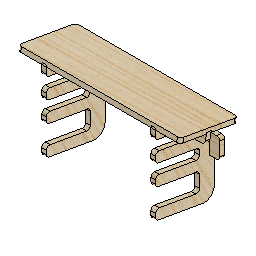
model (Autodesk Fusion 360 design; units mm, degrees)
Autodesk Fusion 360 part; units mm, degrees
note: some values were not read from the file. Set by a fixed rule: which sketch regions a step uses.
sketch "side" plane through (0, 0, 0) normal (1, 0, 0) x (0, 1, 0) in component "mount"
  line L0 (0, 0) -> (0, 102.8022)
  line L1 (0, 102.8022) -> (-75.1927, 116.0607)
  line L2 (-75.1927, 116.0607) -> (-75.1927, 102.8601)
  line L3 (-75.1927, 102.8601) -> (-19, 92.9519)
  line L4 (-19, 92.9519) -> (-19, 79.9519)
  line L5 (-19, 79.9519) -> (-75.1927, 89.8601)
  line L6 (-75.1927, 89.8601) -> (-75.1927, 76.6596)
  line L7 (-75.1927, 76.6596) -> (-19, 66.7513)
  line L8 (-19, 66.7513) -> (-19, 53.7513)
  line L9 (-19, 53.7513) -> (-75.1927, 63.6596)
  line L10 (-75.1927, 63.6596) -> (-75.1927, 50.459)
  line L11 (-75.1927, 50.459) -> (-19, 40.5508)
  line L12 (-19, 40.5508) -> (-19, 16.5508)
  line L13 (-19, 16.5508) -> (-75.1927, 26.459)
  line L14 (-75.1927, 26.459) -> (-75.1927, 13.2585)
  line L15 (-75.1927, 13.2585) -> (0, 0)
  line L16 (-19, 92.9519) -> (0, 92.9519) construction
  line L17 (-74.8454, 115.9994) -> (-75.1927, 114.0298)
  line L18 (-74.8454, 115.9994) -> (-74.1508, 119.9387) construction
  line L19 (-75.1927, 116.0607) -> (-75.1927, 119.9387) construction
  line L20 (-74.1508, 119.9387) -> (-75.1927, 119.9387) construction
  dimension "d9" = 80
  dimension "d14" = 13
  dimension "d15" = 13
  dimension "d16" = 13
  dimension "d21" = 2
  dimension "d33" = 24
  dimension "d43" = 4
  dimension "d44" = 76
  dimension "d53" = 19
  constraint coincident L0.start L15.end
  constraint vertical L0
  constraint parallel L0 L2
  constraint parallel L1 L3
  constraint parallel L0 L4
  constraint coincident L0 L16.end
  constraint perpendicular L0 L16
  constraint collinear L2 L6
  constraint collinear L6 L10
  constraint collinear L10 L14
  constraint collinear L4 L8
  constraint collinear L8 L12
  constraint equal L2 L6
  constraint equal L6 L10
  constraint equal L10 L14
  constraint parallel L5 L7
  constraint parallel L9 L11
  constraint parallel L13 L15
  constraint parallel L3 L5
  constraint parallel L7 L9
  constraint parallel L11 L13
  constraint coincident L1 L17.start
  constraint coincident L2 L17.end
  constraint perpendicular L1 L17
  constraint perpendicular L1 L18
  constraint parallel L2 L19
  constraint perpendicular L19 L20
  measures "d9" angle of L0 L1
  measures "d14" distance of L3.end L4.end
  measures "d15" distance of L1 L3
  measures "d16" distance of L7.end L8.end
  measures "d21" distance of L17.start L17.end
  measures "d33" distance of L11.end L12.end
  measures "d43" distance of L17.start L18.end
  measures "d44" distance of L0.end L17.start
  measures "d53" distance of L0 L4
extrude "Extrude1" add sketch "side" along normal blind 6 contours L0 L1 L2 L3 L4 L5 L6 L7 L8 L9 L10 L11 L12 L13 L14 L15 L17 makes body 1 in component "mount"
copy_body "CopyPasteBodies1" bodies 1 makes body 2 in component "mount"
move_body "Move1" bodies 2 to x (1, 0, 0) y (0, 1, 0) z (0, 0, 1) at (140, 0, 0) in component "mount"
sketch "top" plane through (0, 17.5802, 99.7023) normal (0, 0.173648, 0.984808) x (-1, 0, 0) in component "mount"
  line L0 (0, 17.8514) -> (0, 93.8514)
  line L1 (0, 93.8514) -> (-6, 93.8514)
  line L2 (-6, 93.8514) -> (-6, 17.8514)
  line L3 (-6, 17.8514) -> (0, 17.8514)
  line L4 (31.0081, 18.8514) -> (-176.9919, 18.8514)
  line L5 (-176.9919, 18.8514) -> (-176.9919, 93.8514)
  line L6 (-176.9919, 93.8514) -> (31.0081, 93.8514)
  line L7 (31.0081, 93.8514) -> (31.0081, 18.8514)
  line L8 (-146, 17.8514) -> (-176.9919, 18.8514) construction
  line L9 (31.0081, 56.3514) -> (0, 56.3514) construction
  line L10 (-140, 93.8514) -> (-146, 93.8514)
  line L11 (-146, 93.8514) -> (-146, 17.8514)
  line L12 (-146, 17.8514) -> (-140, 17.8514)
  line L13 (-140, 17.8514) -> (-140, 93.8514)
  line L14 (31.0081, 53.3514) -> (-176.9919, 53.3514)
  line L15 (31.0081, 59.3514) -> (-176.9919, 59.3514)
  line L16 (15.504, 53.3514) -> (15.504, 59.3514) construction
  point P0 (-146, 17.8514)
  point P1 (-140, 93.8514)
  dimension "d23" = 75
  dimension "d24" = 208
  dimension "d40" = 6
  constraint horizontal L4
  constraint vertical L5
  constraint horizontal L6
  constraint vertical L7
  constraint coincident P0 L8.start
  constraint midpoint L7 L9.start
  constraint coincident L0 L9.end
  constraint perpendicular L0 L9
  constraint equal L8 L9
  constraint horizontal L10
  constraint vertical L11
  constraint horizontal L12
  constraint vertical L13
  constraint coincident P1 L10.start
  constraint coincident L7 L14.start
  constraint coincident L5 L14.end
  constraint perpendicular L5 L14
  constraint coincident L7 L15.start
  constraint coincident L5 L15.end
  constraint perpendicular L5 L15
  constraint coincident L14 L16.start
  constraint coincident L15 L16.end
  constraint perpendicular L15 L16
  constraint midpoint L9 L16
  constraint collinear L6 L10
  measures "d23" distance of L4 L6
  measures "d24" distance of L5 L7
  measures "d40" distance of L14 L15
extrude "Extrude5" add sketch "top" against normal up to surface (2 mm away) separate body contours L0 L4 L7 L14 | L2 L4 L13 L14 | L0 L6 L7 L15 | L2 L6 L13 L15 | L4 L5 L11 L14 | L5 L6 L11 L15 makes body 3 at (-20.672, -52.1948, 112.0055) makes body 4 at (-10.336, -12.3101, 104.9728) makes body 5 at (156.3306, -23.6354, 106.9697) makes body 6 at (50.6667, -52.1948, 112.0055) makes body 7 at (50.6667, -12.3101, 104.9728) makes body 8 at (166.6613, -52.1948, 112.0055) in component "mount"
extrude "Extrude6" add sketch "top" along normal blind 4 contours L0 L2 L4 L14 | L0 L4 L7 L14 | L0 L2 L14 L15 | L0 L7 L14 L15 | L2 L4 L13 L14 | L0 L1 L2 L6 L15 | L0 L6 L7 L15 | L2 L13 L14 L15 | L4 L11 L13 L14 | L2 L6 L13 L15 | L11 L13 L14 L15 | L4 L5 L11 L14 | L6 L10 L11 L13 L15 | L5 L11 L14 L15 | L5 L6 L11 L15 bodies 3 4 5 6 7 8 in component "mount"
sketch "notch" plane through (0, 0, 0) normal (-1, 0, 0) x (0, -1, 0) in component "mount"
  line L0 (0, 102.8022) -> (0, 0)
  line L1 (0, 0) -> (75.1927, 13.2585)
  line L2 (75.1927, 13.2585) -> (75.1927, 26.459)
  line L3 (75.1927, 26.459) -> (19, 16.5508)
  line L4 (19, 16.5508) -> (19, 40.5508)
  line L5 (19, 40.5508) -> (75.1927, 50.459)
  line L6 (75.1927, 50.459) -> (75.1927, 63.6596)
  line L7 (75.1927, 63.6596) -> (19, 53.7513)
  line L8 (19, 53.7513) -> (19, 66.7513)
  line L9 (19, 66.7513) -> (75.1927, 76.6596)
  line L10 (75.1927, 76.6596) -> (75.1927, 89.8601)
  line L11 (75.1927, 89.8601) -> (19, 79.9519)
  line L12 (19, 79.9519) -> (19, 92.9519)
  line L13 (19, 92.9519) -> (75.1927, 102.8601)
  line L14 (75.1927, 102.8601) -> (75.1927, 114.0298)
  line L15 (75.1927, 114.0298) -> (74.8454, 115.9994)
  line L16 (74.8454, 115.9994) -> (0, 102.8022)
  line L17 (34.9607, 108.9667) -> (37.2181, 96.1642)
  line L18 (40.8695, 110.0086) -> (43.1269, 97.2061)
  line L19 (34.9607, 108.9667) -> (40.8695, 110.0086)
  line L20 (37.2181, 96.1642) -> (43.1269, 97.2061)
  line L21 (36.0894, 102.5654) -> (41.9982, 103.6073)
  point P0 (35.308, 106.9971)
  point P1 (34.9607, 108.9667)
  point P2 (40.8695, 110.0086)
  point P3 (41.2168, 108.039)
  constraint coincident P1 L17.start
  constraint coincident L13 L17.end
  constraint perpendicular L13 L17
  constraint coincident P2 L18.start
  constraint coincident L13 L18.end
  constraint perpendicular L13 L18
  constraint midpoint L17 L21.start
  constraint midpoint L18 L21.end
extrude "Extrude7" cut sketch "notch" against normal up to surface (146 mm away) contours L16 L17 L18 L19 L21 bodies 1 2 in component "mount"
extrude "Extrude8" add sketch "notch" along normal up to surface (31.0081 mm away) and the other way up to surface (176.9919 mm away) separate body contours L16 L17 L18 L19 L21 | L13 L17 L18 L20 L21 makes body 9 in component "mount"
combine "Combine1" operation cut target body 9 tool bodies 1 2 keep tools in component "mount"
sketch "stretcher" plane through (0, 0, 0) normal (0, 1, 0) x (-1, 0, 0) in component "mount"
  line L0 (-140, 0) -> (-140, 102.8022)
  line L1 (-140, 102.8022) -> (-146, 102.8022)
  line L2 (-146, 102.8022) -> (-146, 0)
  line L3 (-146, 0) -> (-140, 0)
  line L4 (-6, 0) -> (-6, 102.8022)
  line L5 (0, 0) -> (0, 102.8022)
  line L6 (-159, 77.8022) -> (13, 77.8022)
  line L7 (13, 77.8022) -> (13, 51.8022)
  line L8 (13, 51.8022) -> (-159, 51.8022)
  line L9 (-159, 51.8022) -> (-159, 77.8022)
  line L10 (-159, 64.8022) -> (13, 64.8022) construction
  line L11 (-159, 77.8022) -> (-146, 64.8022) construction
  line L12 (0, 64.8022) -> (13, 77.8022) construction
  line L13 (-146, 71.3022) -> (-140, 71.3022)
  line L14 (-146, 51.8022) -> (-146, 58.3022) construction
  line L15 (-140, 58.3022) -> (-146, 58.3022)
  line L16 (-146, 71.3022) -> (-146, 77.8022) construction
  line L17 (-6, 71.3022) -> (0, 71.3022)
  line L18 (-6, 58.3022) -> (0, 58.3022)
  circle A0 centre (-127, 64.8022) radius 2.25
  circle A1 centre (-19, 64.8022) radius 2.25
  line L19 (-140, 77.8022) -> (-127, 64.8022) construction
  line L20 (-6, 77.8022) -> (-19, 64.8022) construction
  point P0 (-140, 64.8022)
  dimension "d61" = 26
  dimension "d62" = 13
  dimension "d63" = 6.5
  dimension "d64" = 25
  dimension "d67" = 4.5
  constraint horizontal L6
  constraint vertical L7
  constraint horizontal L8
  constraint vertical L9
  constraint midpoint L9 L10.start
  constraint midpoint L7 L10.end
  constraint coincident L10 L11.end
  constraint coincident L2 L11.end
  constraint coincident L5 L12.start
  constraint coincident L10 L12.start
  constraint equal L11 L12
  constraint coincident L10 P0
  constraint coincident L2 L13.start
  constraint coincident L0 L13.end
  constraint perpendicular L0 L13
  constraint coincident L8 L14.start
  constraint coincident L2 L14.start
  constraint coincident L2 L14.end
  constraint perpendicular L8 L14
  constraint coincident L0 L15.start
  constraint parallel L8 L15
  constraint coincident L6 L16.end
  constraint coincident L2 L16.end
  constraint equal L14 L16
  constraint coincident L4 L17.start
  constraint coincident L5 L17.end
  constraint perpendicular L5 L17
  constraint coincident L4 L18.start
  constraint coincident L5 L18.end
  constraint perpendicular L5 L18
  constraint collinear L13 L17
  constraint collinear L15 L18
  constraint coincident L10 A0.centre
  constraint coincident L10 A1.centre
  constraint equal A0 A1
  constraint coincident L6 L19.start
  constraint coincident L0 L19.start
  constraint coincident A0.centre L19.end
  constraint coincident L4 L20.start
  constraint coincident L6 L20.start
  constraint coincident A1.centre L20.end
  constraint equal L19 L20
  constraint equal L11 L19
  measures "d61" distance of L6.start L8.end
  measures "d62" distance of L2 L9
  measures "d63" distance of L6 L13
  measures "d64" distance of L1 L6
  measures "d67" diameter of A0
extrude "Extrude9" add sketch "stretcher" against normal blind 6 separate body contours L0 L2 L13 L15 | L0 L4 L6 L8 | L2 L6 L8 L9 | L4 L5 L17 L18 | L5 L6 L7 L8 makes body 10 in component "mount"
combine "Combine2" operation cut target body 2 tool bodies 10 keep tools in component "mount"
combine "Combine3" operation cut target body 1 tool bodies 10 keep tools in component "mount"
fillet "Fillet3" radius 4 36 edges at (3, -75.1927, 102.8601) (3, -75.1927, 13.2585) (3, -75.1927, 26.459) (3, -75.1927, 50.459) (3, -75.1927, 63.6596) (3, -75.1927, 76.6596) (3, -75.1927, 89.8601) (3, -19, 92.9519) (3, -19, 40.5508) (3, -19, 66.7513) (3, -19, 79.9519) (3, -19, 53.7513) (3, -19, 16.5508) (143, -75.1927, 102.8601) (143, -75.1927, 89.8601) (143, -75.1927, 76.6596) (143, -75.1927, 63.6596) (143, -75.1927, 50.459) (143, -75.1927, 26.459) (143, -75.1927, 13.2585) (143, -19, 92.9519) (143, -19, 66.7513) (143, -19, 40.5508) (143, -19, 16.5508) (143, -19, 53.7513) (143, -19, 79.9519) (-31.0081, -0.8112, 103.9606) (-31.0081, -74.6717, 116.9843) (176.9919, -74.6717, 116.9843) (176.9919, -0.8112, 103.9606) (-31.0081, -40.1725, 96.6851) (176.9919, -40.1725, 96.6851) (159, -3, 77.8022) (159, -3, 51.8022) (-13, -3, 77.8022) (-13, -3, 51.8022) on bodies 1 2 3 9 10 in component "mount"
fillet "Fillet3" radius 13 2 edges at (3, 0, 0) (143, 0, 0) on bodies 1 2 3 9 10 in component "mount"
component "mount" placed x (1, 0, 0) y (0, 1, 0) z (0, 0, 1) at (0, 0, 0)
equation "plateWidth = 76 mm"
equation "plateThickness = 10 mm"
equation "plateLength = 203 mm"
equation "stropWidth = 64 mm"
equation "stropThickness = 21 mm"
equation "stropLength = 203 mm"
equation "stockThickness = 6 mm"
equation "d9 = 90 deg - angle"
equation "angle = 10 deg"
equation "d14 = d16"
equation "d15 = memberWidth"
equation "d16 = plateThickness + 3 mm"
equation "d17 = stockThickness"
equation "d21 = overlap"
equation "d23 = topDepth"
equation "d24 = topWidth"
equation "overlap = stockThickness / 3"
equation "d33 = stropThickness + 3 mm"
equation "d40 = stockThickness"
equation "topWidth = 208 mm"
equation "topDepth = 75 mm"
equation "d43 = stockThickness - d21"
equation "d44 = topDepth + 1 mm"
equation "d49 = stockThickness - overlap"
equation "memberWidth = 13 mm"
equation "spineWidth = 13 mm + stockThickness"
equation "d53 = spineWidth"
equation "d61 = 2 * memberWidth"
equation "d62 = memberWidth"
equation "d63 = memberWidth / 2"
equation "d65 = -stockThickness"
